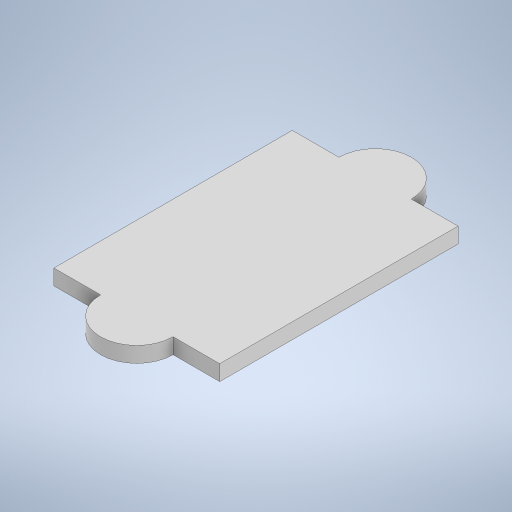
# Autodesk Inventor part: external_input
Saved by Autodesk Inventor 2024.1 (Build 281209000, 209)
## iProperties
Created: 2025-04-13
Part Number: external_input
Material: 一般
Document SubType Name: Modeling
Designer: hibik
Density: 1 g/cm^3
Appearance: 既定
Author: hibik
Autodesk Inventor part; units mm, degrees
ref_plane "YZ Plane" through (0, 0, 0) normal (1, 0, 0) x (0, 1, 0)
ref_plane "XZ Plane" through (0, 0, 0) normal (0, 1, 0) x (-1, 0, 0)
ref_plane "XY Plane" through (0, 0, 0) normal (0, 0, 1) x (1, 0, 0)
sketch "スケッチ1" plane through (0, 0, 0) normal (0, 1, 0) x (-1, 0, 0)
  line L0 (0, 0) -> (16, 0)
  line L1 (16, 0) -> (16, -30)
  line L2 (16, -30) -> (0, -30)
  line L3 (0, -30) -> (0, 0)
  circle A0 centre (8, -3.5) radius 3.5
  circle A1 centre (8, -26.5) radius 3.5
  line L4 (16, -3.5) -> (0, -3.5)
  line L5 (16, -26.5) -> (-0.2656, -26.5)
  point P0 (8, 0)
  point P1 (11.5, -3.5)
  point P2 (4.5, -3.5)
  point P3 (0, -26.5)
  point P4 (4.5, -26.5)
  point P5 (11.5, -26.5)
  dimension "d0" = 16
  dimension "d1" = 30
  dimension "d2" = 7
  constraints: 12 end point, 4 point on line, 3 perpendicular, 2 centre point, 2 midpoint, 2 parallel, 2 tangent, 2 vertical alignment, 1 equal radius, 1 horizontal
  measures "d0" distance of L1.end L2.end
  measures "d1" distance of L0.end L1.end
  measures "d2" diameter of A0
extrude "押し出し1" add sketch "スケッチ1" along normal blind 1.5 contours A0 L4 | L4 A0 L1 L5 A1 L3 | A0 L4 | L5 A1 | A1 L5
